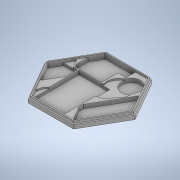
# Autodesk Inventor part: Factions_Base
Saved by Autodesk Inventor 2021 (Build 250183000, 183)
## iProperties
Created: 2023-03-16
Part Number: Factions_Base
Material: ABS Plastic
Document SubType Name: Modeling
Designer: Bradley
Density: 1.06 g/cm^3
Appearance: Smooth - Medium Gray
Author: Bradley
Autodesk Inventor part; units mm, degrees
ref_plane "YZ Plane" through (0, 0, 0) normal (1, 0, 0) x (0, 1, 0)
ref_plane "XZ Plane" through (0, 0, 0) normal (0, 1, 0) x (-1, 0, 0)
ref_plane "XY Plane" through (0, 0, 0) normal (0, 0, 1) x (1, 0, 0)
sketch "Sketch1" plane through (0, 0, 0) normal (0, 1, 0) x (-1, 0, 0)
  line L0 (-29.4449, -51) -> (-58.8897, 0)
  line L1 (-58.8897, 0) -> (-29.4449, 51)
  line L2 (-29.4449, 51) -> (29.4449, 51)
  line L3 (29.4449, 51) -> (58.8897, 0)
  line L4 (58.8897, 0) -> (29.4449, -51)
  line L5 (29.4449, -51) -> (-29.4449, -51)
  line L6 (-31.2924, -54.2) -> (-62.5848, 0)
  line L7 (-62.5848, 0) -> (-31.2924, 54.2)
  line L8 (-31.2924, 54.2) -> (31.2924, 54.2)
  line L9 (31.2924, 54.2) -> (62.5848, 0)
  line L10 (62.5848, 0) -> (31.2924, -54.2)
  line L11 (31.2924, -54.2) -> (-31.2924, -54.2)
  line L12 (-30.3109, -52.5) -> (-60.6218, 0)
  line L13 (-60.6218, 0) -> (-30.3109, 52.5)
  line L14 (-30.3109, 52.5) -> (30.3109, 52.5)
  line L15 (30.3109, 52.5) -> (60.6218, 0)
  line L16 (60.6218, 0) -> (30.3109, -52.5)
  line L17 (30.3109, -52.5) -> (-30.3109, -52.5)
  line L18 (-30.4264, -52.7) -> (-60.8527, 0)
  line L19 (-60.8527, 0) -> (-30.4264, 52.7)
  line L20 (-30.4264, 52.7) -> (30.4264, 52.7)
  line L21 (30.4264, 52.7) -> (60.8527, 0)
  line L22 (60.8527, 0) -> (30.4264, -52.7)
  line L23 (30.4264, -52.7) -> (-30.4264, -52.7)
  line L24 (0, -51) -> (0, -52.5) construction
  line L25 (0, -52.7) -> (0, -54.2) construction
  line L26 (28.9449, 50.5) -> (-13.0551, 50.5) construction
  line L27 (-13.0551, 50.5) -> (-13.0551, -13.5) construction
  line L28 (-13.0551, -13.5) -> (28.9449, -13.5) construction
  line L29 (28.9449, -13.5) -> (28.9449, 50.5) construction
  line L30 (29.4449, -14) -> (-13.5551, -14)
  line L31 (-13.5551, -14) -> (-13.5551, 51)
  line L32 (-13.5551, 51) -> (29.4449, 51)
  line L33 (29.4449, 51) -> (29.4449, -14)
  line L34 (-13.8231, 27.4577) -> (-42.4597, 27.4577) construction
  line L35 (-42.4597, 27.4577) -> (-28.1414, 52.2577) construction
  line L36 (-28.1414, 52.2577) -> (-13.8231, 27.4577) construction
  line L37 (-15.5551, 30.4577) -> (-17.2872, 27.4577) construction
  line L38 (-15.0551, 51) -> (-15.0551, -15.5)
  line L39 (-15.0551, -15.5) -> (30.9449, -15.5)
  line L40 (30.9449, -15.5) -> (30.9449, 48.4019)
  circle A0 centre (21.8671, 37.875) radius 13.125 construction
  circle A1 centre (21.8671, 37.875) radius 12.625 construction
  circle A2 centre (13.0949, 34.65) radius 15.85 construction
  circle A3 centre (2.7949, 3.6145) radius 16.35 construction
  circle A4 centre (13.0949, 34.65) radius 16.35 construction
  line L41 (58.168, -0.25) -> (43.8498, -25.05) construction
  line L42 (43.8498, -25.05) -> (29.5315, -0.25) construction
  line L43 (29.5315, -0.25) -> (58.168, -0.25) construction
  line L44 (32.9956, -0.25) -> (31.2635, -3.25) construction
  line L45 (29.5315, -0.25) -> (44.2828, 25.3) construction
  line L46 (30.9449, -3.6981) -> (30.4449, -2.8321)
  line L47 (30.4449, -2.8321) -> (30.4449, 2.3321)
  line L48 (30.4449, 2.3321) -> (30.9449, 3.1981)
  line L49 (30.9449, 3.1981) -> (43.9941, 25.8)
  line L50 (37.8164, -16.6) -> (25.3164, -16.6) construction
  line L51 (25.3164, -16.6) -> (25.3164, -37.5) construction
  line L52 (25.3164, -37.5) -> (37.8164, -37.5) construction
  line L53 (37.8164, -37.5) -> (37.8164, -16.6) construction
  line L54 (35.8164, -37.5) -> (37.8164, -35.5) construction
  line L55 (37.8164, -37.5) -> (37.8164, -35.5) construction
  line L56 (27.3164, -16.6) -> (25.3164, -18.6) construction
  circle A5 centre (37.8164, -35.5) radius 0.5 construction
  circle A6 centre (35.8164, -37.5) radius 0.5 construction
  line L57 (24.8164, -36.9) -> (12.3164, -36.9) construction
  line L58 (12.3164, -36.9) -> (12.3164, -16) construction
  line L59 (12.3164, -16) -> (24.8164, -16) construction
  line L60 (24.8164, -16) -> (24.8164, -36.9) construction
  line L61 (8.9109, -50.5) -> (-11.9891, -50.5) construction
  line L62 (-11.9891, -50.5) -> (-11.9891, -38) construction
  line L63 (-11.9891, -38) -> (8.9109, -38) construction
  line L64 (8.9109, -38) -> (8.9109, -50.5) construction
  line L65 (-1.1836, -15.5) -> (-1.1836, -37.5)
  line L66 (-1.1836, -37.5) -> (-12.4891, -37.5)
  circle A7 centre (-25.7027, -31.2317) radius 12.625 construction
  line L67 (-26.4093, 49.2577) -> (-29.8734, 49.2577) construction
  circle A8 centre (16.3199, 3.811) radius 13.125 construction
  line L68 (-13.8231, 26.9577) -> (-42.4597, 26.9577) construction
  line L69 (-42.4597, 26.9577) -> (-28.1414, 2.1577) construction
  line L70 (-28.1414, 2.1577) -> (-13.8231, 26.9577) construction
  line L71 (-28.5744, 1.9077) -> (-42.8927, 26.7077) construction
  line L72 (-42.8927, 26.7077) -> (-57.211, 1.9077) construction
  line L73 (-57.211, 1.9077) -> (-28.5744, 1.9077) construction
  line L74 (-30.4885, 1.4077) -> (-44.8068, -23.3923) construction
  line L75 (-44.8068, -23.3923) -> (-59.1251, 1.4077) construction
  line L76 (-59.1251, 1.4077) -> (-30.4885, 1.4077) construction
  line L77 (-55.661, 1.4077) -> (-57.3931, -1.5923) construction
  circle A9 centre (-25.7027, -31.2317) radius 14.625 construction
  circle A10 centre (-25.7027, -31.2317) radius 6.7683 construction
  line L78 (-15.0551, 23.8237) -> (-43.8498, -26.05)
  circle A11 centre (-25.7027, -31.2317) radius 13.125
  circle A12 centre (-0.4301, 24.0224) radius 13.125 construction
  circle A13 centre (-14.4766, -7.5032) radius 13.125 construction
  line L79 (52.3449, -12.75) -> (31.4449, -12.75) construction
  line L80 (31.4449, -12.75) -> (31.4449, -0.25) construction
  line L81 (31.4449, -0.25) -> (52.3449, -0.25) construction
  line L82 (52.3449, -0.25) -> (52.3449, -12.75) construction
  line L83 (50.3449, -12.75) -> (52.3449, -10.75) construction
  line L84 (30.9449, -15.5) -> (49.9408, -15.5)
  line L85 (30.9449, -14) -> (50.8068, -14)
  line L86 (37.7587, -15.5) -> (43.8498, -26.05)
  line L87 (35.8164, -16.6) -> (37.8164, -18.6) construction
  line L88 (36.0267, -15.5) -> (42.9837, -27.55)
  line L89 (30.3109, -50.5) -> (9.4109, -50.5) construction
  line L90 (9.4109, -50.5) -> (9.4109, -38) construction
  line L91 (9.4109, -38) -> (30.3109, -38) construction
  line L92 (30.3109, -38) -> (30.3109, -50.5) construction
  line L93 (28.3109, -50.5) -> (30.3109, -48.5) construction
  circle A14 centre (28.3109, -50.5) radius 0.5 construction
  circle A15 centre (30.3109, -48.5) radius 0.5 construction
  line L94 (-12.4891, -37.5) -> (-12.4891, -51)
  line L95 (11.8164, -36.9) -> (-0.6836, -36.9) construction
  line L96 (-0.6836, -36.9) -> (-0.6836, -16) construction
  line L97 (-0.6836, -16) -> (11.8164, -16) construction
  line L98 (11.8164, -16) -> (11.8164, -36.9) construction
  circle A16 centre (-19.7736, -20.0488) radius 16.35 construction
  circle A17 centre (-19.7736, -20.0488) radius 17.85 construction
  circle A18 centre (-14.4766, -7.5032) radius 14.625 construction
  line L99 (-26.8379, 51) -> (-15.0551, 30.5917)
  line L100 (-32.812, -42.2644) -> (-34.0693, -42.9903)
  line L101 (-38.812, -31.8721) -> (-40.0693, -32.598)
  line L102 (38.3164, -19.466) -> (38.3164, -35.634)
  point P0 (0, 0)
  point P1 (0, 0)
  point P2 (0, 0)
  point P3 (-13.5551, 51)
  point P4 (-4.0691, -15.5)
  point P5 (-37.0693, -37.7942)
  dimension "d0" = 102
  dimension "d2" = 0.2
  dimension "d16" = 108.4
  dimension "d17" = 42
  dimension "d18" = 64
  dimension "d19" = 43
  dimension "d21" = 24.8
  dimension "d22" = 21.8
  dimension "d26" = 65
  dimension "d27" = 1.5
  dimension "d28" = 1.5
  dimension "d29" = 1.5
  dimension "d36" = 25.25
  dimension "d37" = 0.5
  dimension "d38" = 31.7
  dimension "d39" = 0.5
  dimension "d41" = 24.8
  dimension "d42" = 21.8
  dimension "d43" = 0.5
  dimension "d44" = 1
  dimension "d45" = 0.5
  dimension "d46" = 0.25
  dimension "d47" = 0.5
  dimension "d50" = 35.5
  dimension "d54" = 45
  dimension "d55" = 2
  dimension "d56" = 1
  dimension "d67" = 0.5
  dimension "d74" = 0.5
  dimension "d77" = 0.5
  dimension "d78" = 0.5
  dimension "d79" = 0.5
  dimension "d80" = 0.5
  dimension "d81" = 0.5
  dimension "d84" = 0.5
  dimension "d85" = 1.5
  dimension "d86" = 45
  dimension "d87" = 2
  dimension "d88" = 12.5
  dimension "d89" = 20.9
  dimension "d90" = 0.5
  dimension "d91" = 1.5
  dimension "d92" = 0.5
  dimension "d93" = 0.5
  dimension "d94" = 0.5
  dimension "d95" = 0.5
  dimension "d96" = 0.5
  dimension "d97" = 0.5
  dimension "d98" = 0.5
  dimension "d99" = 0.5
  dimension "d100" = 0.5
  dimension "d102" = 1.5
  dimension "d103" = 0.5
  dimension "d107" = 6
  dimension "d108" = 6
  dimension "d109" = 0.5
  constraints: 207 end point, 43 point on line, 37 parallel, 23 equal length, 16 centre point, 13 coincident, 13 horizontal, 13 tangent, 12 perpendicular, 10 equal radius, 9 collinear, 4 midpoint, 3 vertical, 2 point on circle, 1 vertical alignment, 45 other
  measures "d0" distance between parallel lines of L2 L5
  measures "d2" distance between parallel lines of L17 L23
  measures "d16" distance between parallel lines of L8 L11
  measures "d17" distance of L27.end L28.end
  measures "d18" distance of L26.end L27.end
  measures "d19" distance between parallel lines of L31 L33
  measures "d21" distance from line of L35.end L34
  measures "d22" distance between parallel lines of L35 L37
  measures "d26" distance of L2.end L30.start
  measures "d27" distance between parallel lines of L39 L30
  measures "d28" distance between parallel lines of L38 L31
  measures "d29" distance between parallel lines of L33 L40
  measures "d36" diameter of A1
  measures "d37" radial gap between concentric circles of A1 A0
  measures "d38" diameter of A2
  measures "d39" radial gap between concentric circles of A4 A2
  measures "d41" distance from line of L42.end L41
  measures "d42" distance between parallel lines of L44 L41
  measures "d43" distance between parallel lines of L41 L4
  measures "d44" distance between parallel lines of L33 L47
  measures "d45" distance between parallel lines of L42 L46
  measures "d46" distance from line of L3.end L43
  measures "d47" distance between parallel lines of L45 L48
  measures "d50" distance between parallel lines of L39 L5
  measures "d54" angle of L55 L54
  measures "d55" distance of L52.end L54.end
  measures "d56" diameter of A6
  measures "d67" distance between parallel lines of L39 L59
  measures "d74" distance between parallel lines of L1 L35
  measures "d77" distance from line of L37.start L38
  measures "d78" distance between parallel lines of L34 L68
  measures "d79" distance between parallel lines of L71 L69
  measures "d80" distance between parallel lines of L73 L76
  measures "d81" distance between parallel lines of L0 L75
  measures "d84" distance between parallel lines of L78 L70
  measures "d86" angle of L83 L79
  measures "d87" horizontal distance of L83.start L83.end
  measures "d88" distance of L81.end L79.start
  measures "d89" distance of L79.start L79.end
  measures "d90" distance between parallel lines of L40 L80
  measures "d91" distance between parallel lines of L88 L86
  measures "d92" distance between parallel lines of L60 L51
  measures "d93" distance between parallel lines of L5 L89
  measures "d94" distance between parallel lines of L52 L91
  measures "d95" distance between parallel lines of L64 L90
  measures "d96" distance between parallel lines of L94 L62
  measures "d97" distance between parallel lines of L98 L58
  measures "d98" distance between parallel lines of L65 L96
  measures "d99" distance between parallel lines of L63 L66
  measures "d100" radial gap between concentric circles of A4 A2
  measures "d103" distance between parallel lines of L36 L99
  measures "d107" distance from line of L100 A7.centre
  measures "d108" distance from line of L101 A7.centre
  measures "d109" distance between parallel lines of L53 L102
extrude "Extrusion1" add sketch "Sketch1" against normal blind 1 contours L0 L100 A11 L101 L78 L38 L39 L65 L66 L94 L5 | L0 A11 L100 | L94 L66 L65 L39 L84 L88 L102 L4 L5 | L0 L101 A11 | A11 | L102 L88 L4 | L0 L1 L2 L99 L38 L78 | L88 L84 L86 L4 | L39 L38 L2 L31 L30 L33 L3 L40 L48 L47 L46 | L86 L84 L4 | L84 L40 L85 L4 | L99 L2 L38 | L40 L49 L3 L4 L85 | L46 L47 L48 L40 | L2 L33 L30 L31 | L40 L3 L49 | L6 L7 L8 L9 L10 L11 | L12 L13 L14 L15 L16 L17 | L18 L19 L20 L21 L22 L23
extrude "Extrusion2" add sketch "Sketch1" along normal blind 7.5 contours L12 L13 L14 L15 L16 L17
extrude "Extrusion3" add sketch "Sketch1" along normal blind 4.5 contours L6 L7 L8 L9 L10 L11 | L18 L19 L20 L21 L22 L23
extrude "Extrusion4" add sketch "Sketch1" along normal blind 5.5 contours L0 L100 A11 L101 L78 L38 L39 L65 L66 L94 L5 | L102 L88 L4 | L88 L84 L86 L4 | L39 L38 L2 L31 L30 L33 L3 L40 L48 L47 L46 | L86 L84 L4 | L84 L40 L85 L4 | L99 L2 L38 | L46 L47 L48 L40 | L40 L3 L49
sketch "Sketch2" plane through (0, 5.5, 0) normal (0, 1, 0) x (1, 0, 0)
  line L0 (-37.7587, 15.5) -> (-43.8498, 26.05) projected
  line L1 (13.5551, 14) -> (13.5551, -51) projected
  line L2 (26.8379, -51) -> (13.5551, -51) projected
  line L3 (26.8379, -51) -> (15.0551, -30.5917) projected
  line L4 (15.0551, -30.5917) -> (15.0551, -23.8237) projected
  line L5 (15.0551, -23.8237) -> (43.8498, 26.05) projected
  line L6 (29.4449, 51) -> (34.0693, 42.9903) projected
  arc A0 (32.812, 42.2644) -> (38.812, 31.8721) centre (25.7027, 31.2317) ccw projected
  line L7 (40.0693, 32.598) -> (43.8498, 26.05) projected
  line L8 (12.4891, 51) -> (29.4449, 51) projected
  line L9 (12.4891, 51) -> (12.4891, 37.5) projected
  line L10 (12.4891, 37.5) -> (1.1836, 37.5) projected
  line L11 (1.1836, 37.5) -> (1.1836, 15.5) projected
  line L12 (1.1836, 15.5) -> (-36.0267, 15.5) projected
  line L13 (-36.0267, 15.5) -> (-38.3164, 19.466) projected
  line L14 (-50.8068, 14) -> (-38.3164, 35.634) projected
  line L15 (-50.8068, 14) -> (-30.9449, 14) projected
  line L16 (-30.9449, 14) -> (-30.9449, -3.1981) projected
  line L17 (-30.9449, -3.1981) -> (-43.9941, -25.8) projected
  line L18 (-29.4449, -51) -> (-43.9941, -25.8) projected
  line L19 (-29.4449, -51) -> (-29.4449, 14) projected
  line L20 (-29.4449, 14) -> (13.5551, 14) projected
  circle A1 centre (14.4766, 7.5032) radius 13.125 construction
  circle A2 centre (19.7736, 20.0488) radius 16.35 construction
  circle A3 centre (-21.8671, -37.875) radius 13.125 construction
  line L21 (-37.7587, 15.5) -> (-36.8927, 14)
  line L22 (-50.8068, 14) -> (-30.9449, 14) projected
  line L23 (-29.4449, 14) -> (13.5551, 14) construction
  arc A4 (4.0691, 15.5) -> (3.0724, 14) centre (14.4766, 7.5032) ccw
  arc A5 (32.812, 42.2644) -> (38.812, 31.8721) centre (25.7027, 31.2317) ccw construction
  arc A6 (13.1263, 34.9866) -> (4.0691, 15.5) centre (19.7736, 20.0488) ccw
  arc A7 (27.4661, 5.6215) -> (35.8679, 22.929) centre (19.7736, 20.0488) ccw
  arc A8 (13.5551, -5.5894) -> (27.4661, 5.6215) centre (14.4766, 7.5032) ccw
  line L24 (-29.4449, -51) -> (-29.4449, 14) projected
  arc A9 (-29.4449, -27.1585) -> (-34.9765, -38.5155) centre (-21.8671, -37.875) ccw
  line L25 (-29.4449, -51) -> (-43.9941, -25.8) projected
  line L26 (-36.2337, -39.2413) -> (-34.9765, -38.5155)
  line L27 (40.0693, 32.598) -> (38.812, 31.8721) projected
  line L28 (32.812, 42.2644) -> (34.0693, 42.9903) projected
  line L29 (-38.3164, 19.466) -> (-38.3164, 35.634) projected
  point P0 (0, 0)
  point P1 (37.0693, 37.7942)
  point P2 (13.1263, 34.9866)
  point P3 (3.0724, 14)
  dimension "d104" = 6
  constraints: 22 point on circle, 5 centre point, 5 concentric, 5 point on line, 4 end point, 1 collinear, 1 perpendicular
  measures "d104" distance from line of L26 A3.centre
extrude "Extrusion5" cut sketch "Sketch2" against normal blind 2 contours L21 L15 L14 L0 | L26 A9 L19 L18 | A4 A6 A0 A7 A8 L1 L20
fillet "Fillet2" radius 1 24 edges at (-60.6218, 6, 0) (-30.3109, 6, -52.5) (-30.3109, 6, 52.5) (30.3109, 6, 52.5) (60.6218, 6, 0) (30.3109, 6, -52.5) (-36.8927, 4.5, -14) (-34.9765, 4.5, 38.5155) (-29.4449, 4.5, 27.1585) (3.0724, 4.5, -14) (4.0691, 4.5, -15.5) (13.1263, 4.5, -34.9866) (32.812, 2.75, -42.2644) (1.1836, 2.75, -37.5) (38.812, 2.75, -31.8721) (35.8679, 4.5, -22.929) (27.4661, 4.5, -5.6215) (13.5551, 4.5, 5.5894) (-62.5848, 1.75, 0) (-31.2924, 1.75, 54.2) (31.2924, 1.75, 54.2) (62.5848, 1.75, 0) (31.2924, 1.75, -54.2) (-31.2924, 1.75, -54.2)
fillet "Fillet2" radius 1.5 3 edges at (43.8498, 2.75, -26.05) (-43.9941, 2.75, 25.8) (-43.8498, 4.5, -26.05)
fillet "Fillet2" radius 1 23 edges at (-58.8897, 3.75, 0) (-50.8068, 1.75, -14) (-30.9449, 2.75, -14) (-30.9449, 2.75, 3.1981) (-29.4449, 2.75, -14) (-38.3164, 2.75, -35.634) (-29.4449, 3.75, -51) (12.4891, 2.75, -51) (12.4891, 2.75, -37.5) (1.1836, 2.75, -15.5) (13.5551, 1.75, -14) (34.0693, 2.75, -42.9903) (40.0693, 2.75, -32.598) (15.0551, 2.75, 23.8237) (15.0551, 2.75, 30.5917) (13.5551, 2.75, 51) (-36.2337, 4.5, 39.2413) (-29.4449, 1.75, 51) (26.8379, 2.75, 51) (29.4449, 3.75, 51) (58.8897, 3.75, 0) (29.4449, 6.5, -51) (-29.4449, 5.5, 51)
equation "\"d0\" = Inside"
equation "\"d2\" = Clearance"
equation "\"d16\" = Outside"
equation "\"d17\" = CardWidth"
equation "\"d18\" = CardLength"
equation "\"d19\" = CardWidth + ComponentClearance"
equation "\"d21\" = TriangleHeight"
equation "\"d22\" = TriangleTrimmed"
equation "\"d27\" = DividerThickness"
equation "\"d28\" = d27"
equation "\"d29\" = d27"
equation "\"d8\" = FaceThickness"
equation "\"d10\" = TrayDepth + HexDepth"
equation "\"d30\" = HexDepth + TrayDepth - LidDepth"
equation "\"d32\" = TrayDepth"
equation "\"DividerThickness\" = 1.5"
equation "\"ComponentClearance\" = 1"
equation "\"TrayDepth\" = 5.5"
equation "\"HexDepth\" = 2"
equation "\"Inside\" = 102"
equation "\"Clearance\" = 0.2"
equation "\"Outside\" = 108.4"
equation "\"CardWidth\" = 42"
equation "\"CardLength\" = 64"
equation "\"TriangleHeight\" = 24.8"
equation "\"TriangleTrimmed\" = 21.8"
equation "\"FaceThickness\" = 1"
equation "\"LidDepth\" = 3"
body "Solid1"
